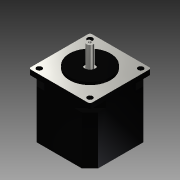
# Autodesk Inventor part: stepper
Saved by Autodesk Inventor 2015 SP1 (Build 190203100, 203)
## iProperties
Created: 2015-03-24
Part Number: stepper
Material: Ogólny
Document SubType Name: Modeling
Designer: Marcin
Density: 1 g/cm^3
Appearance: Gładki - czarny
Author: Marcin
Autodesk Inventor part; units mm, degrees
ref_plane "YZ Plane" through (0, 0, 0) normal (1, 0, 0) x (0, 1, 0)
ref_plane "XZ Plane" through (0, 0, 0) normal (0, 1, 0) x (-1, 0, 0)
ref_plane "XY Plane" through (0, 0, 0) normal (0, 0, 1) x (1, 0, 0)
sketch "Szkic1" plane through (0, 0, 0) normal (0, 0, 1) x (1, 0, 0)
  line L0 (-28.5, -28.5) -> (28.5, -28.5)
  line L1 (28.5, -28.5) -> (28.5, 28.5)
  line L2 (28.5, 28.5) -> (-28.5, 28.5)
  line L3 (-28.5, 28.5) -> (-28.5, -28.5)
  line L4 (-28.5, -28.5) -> (28.5, 28.5) construction
  line L5 (28.5, -28.5) -> (-28.5, 28.5) construction
  line L6 (-28.5, 20.9975) -> (-20.9975, 28.5)
  line L7 (20.9975, 28.5) -> (28.5, 20.9975)
  line L8 (28.5, -20.9975) -> (20.9975, -28.5)
  line L9 (-20.9975, -28.5) -> (-28.5, -20.9975)
  line L10 (0, 32.5269) -> (0, -32.5269) construction
  point P0 (0, 0)
  dimension "d0" = 57
  dimension "d3" = 70
  dimension "d4" = 70
  constraints: 22 end point, 8 point on line, 4 parallel, 3 midpoint, 3 perpendicular, 1 horizontal, 2 other
  measures "d0" distance of L0.end L1.end
  measures "d3" distance between parallel lines of L6 L8
  measures "d4" distance between parallel lines of L7 L9
extrude "Wyciągnięcie proste1" add sketch "Szkic1" along normal blind 45 contours L9 L3 L6 L2 L7 L1 L8 L0
sketch "Szkic2" plane through (0, 0, 45) normal (0, 0, 1) x (1, 0, 0)
  line L0 (20.9975, -28.5) -> (28.5, -20.9975) projected
  line L1 (28.5, -20.9975) -> (28.5, 20.9975) projected
  line L2 (28.5, 20.9975) -> (20.9975, 28.5) projected
  line L3 (20.9975, 28.5) -> (-20.9975, 28.5) projected
  line L4 (-20.9975, 28.5) -> (-28.5, 20.9975) projected
  line L5 (-28.5, 20.9975) -> (-28.5, -20.9975) projected
  line L6 (-28.5, -20.9975) -> (-20.9975, -28.5) projected
  line L7 (-20.9975, -28.5) -> (20.9975, -28.5) projected
  line L8 (20.9975, 28.5) -> (-20.9975, 28.5) projected
  line L9 (13.9264, 28.5) -> (28.5, 13.9264)
  line L10 (28.5, -20.9975) -> (28.5, 20.9975) projected
  line L11 (13.9264, -28.5) -> (28.5, -13.9264)
  line L12 (-20.9975, -28.5) -> (20.9975, -28.5) projected
  line L13 (-13.9264, -28.5) -> (-28.5, -13.9264)
  line L14 (-28.5, 20.9975) -> (-28.5, -20.9975) projected
  line L15 (-28.5, 13.9264) -> (-13.9264, 28.5)
  line L16 (-28.5, -20.9975) -> (-20.9975, -28.5) construction
  line L17 (-24.7487, -24.7487) -> (24.7487, 24.7487) construction
  line L18 (20.9975, -28.5) -> (28.5, -20.9975) construction
  line L19 (24.7487, -24.7487) -> (-24.7487, 24.7487) construction
  line L20 (-20.9975, 28.5) -> (-28.5, 20.9975) construction
  line L21 (-28.5, -20.9975) -> (-20.9975, -28.5) construction
  line L22 (28.5, 20.9975) -> (20.9975, 28.5) construction
  point P0 (0, 0)
  dimension "d7" = 60
  dimension "d8" = 60
  constraints: 12 end point, 8 point on line, 4 midpoint, 4 parallel, 2 other
  measures "d7" distance between parallel lines of L15 L11
  measures "d8" distance between parallel lines of L13 L9
extrude "Wyciągnięcie proste2" add sketch "Szkic2" along normal blind 6 contours L7 L13 L5 L15 L3 L9 L1 L11
sketch "Szkic3" plane through (0, 0, 51) normal (0, 0, 1) x (1, 0, 0)
  line L0 (20.9975, -28.5) -> (28.5, -20.9975) projected
  line L1 (-20.9975, -28.5) -> (20.9975, -28.5) projected
  line L2 (-28.5, -20.9975) -> (-20.9975, -28.5) projected
  line L3 (-28.5, 20.9975) -> (-28.5, -20.9975) projected
  line L4 (-20.9975, 28.5) -> (-28.5, 20.9975) projected
  line L5 (20.9975, 28.5) -> (-20.9975, 28.5) projected
  line L6 (28.5, 20.9975) -> (20.9975, 28.5) projected
  line L7 (28.5, -20.9975) -> (28.5, 20.9975) projected
  line L8 (-28.5, -28.5) -> (28.5, -28.5)
  line L9 (28.5, -28.5) -> (28.5, 28.5)
  line L10 (28.5, 28.5) -> (-28.5, 28.5)
  line L11 (-28.5, 28.5) -> (-28.5, -28.5)
  point P0 (0, 0)
  point P1 (0, 28.5)
  point P2 (28.5, 0)
  point P3 (0, -28.5)
  constraints: 8 end point, 6 midpoint, 2 parallel, 2 perpendicular, 1 horizontal
extrude "Wyciągnięcie proste3" add sketch "Szkic3" along normal blind 4.8
sketch "Szkic4" plane through (0, 0, 55.8) normal (0, 0, 1) x (1, 0, 0)
  circle A0 centre (0, 0) radius 19.05
  dimension "d13" = 38.1
  constraints: 1 centre point, 1 coincident
  measures "d13" diameter of A0
extrude "Wyciągnięcie proste4" add sketch "Szkic4" along normal blind 2.5
sketch "Szkic5" plane through (0, 0, 55.8) normal (0, 0, 1) x (1, 0, 0)
  line L0 (-23.57, -23.57) -> (23.57, -23.57) construction
  line L1 (23.57, -23.57) -> (23.57, 23.57) construction
  line L2 (23.57, 23.57) -> (-23.57, 23.57) construction
  line L3 (-23.57, 23.57) -> (-23.57, -23.57) construction
  line L4 (-23.57, -23.57) -> (23.57, 23.57) construction
  line L5 (23.57, -23.57) -> (-23.57, 23.57) construction
  point P0 (0, 0)
  dimension "d16" = 47.14
  constraints: 12 end point, 4 coincident, 2 midpoint, 2 parallel, 2 perpendicular, 1 horizontal
  measures "d16" distance of L0.end L1.end
hole "Otwór1" at (-23.57, 23.57, 55.8) at (23.57, 23.57, 55.8) at (23.57, -23.57, 55.8) at (-23.57, -23.57, 55.8) direction (0, 0, -1) diameter 5 depth 5
sketch "Szkic6" plane through (0, 0, 58.3) normal (0, 0, 1) x (1, 0, 0)
  circle A0 centre (0, 0) radius 5
  dimension "d24" = 10
  constraints: 1 centre point, 1 coincident
  measures "d24" diameter of A0
extrude "Wyciągnięcie proste5" cut sketch "Szkic6" against normal up to surface (2.5 mm away)
sketch "Szkic7" plane through (0, 0, 55.8) normal (0, 0, 1) x (1, 0, 0)
  circle A0 centre (0, 0) radius 5 projected
  circle A1 centre (0, 0) radius 3.175
  dimension "d27" = 6.35
  constraints: 1 centre point, 1 coincident
  measures "d27" diameter of A1
extrude "Wyciągnięcie proste6" add sketch "Szkic7" along normal blind 21 contours A1
sketch "Szkic8" plane through (0, 0, 76.8) normal (0, 0, 1) x (1, 0, 0)
  circle A0 centre (0, 0) radius 3.175 projected
  line L0 (-2.4659, 2) -> (2.4659, 2)
  dimension "d30" = 2
  constraints: 2 end point, 2 point on circle, 1 horizontal
  measures "d30" distance from line of L0 A0.centre
extrude "Wyciągnięcie proste7" cut sketch "Szkic8" against normal blind 19 contours L0 A0 picked at (-0.6547, 2.1648)
sketch "Szkic9" plane through (0, 0, 76.8) normal (0, 0, 1) x (1, 0, 0)
  point P0 (0, 0)
  point P1 (0, 0)
  constraints: 1 coincident
hole "Otwór2" at (0, 0, 76.8) direction (0, 0, -1) diameter 2.5 depth 2 tip angle 118
fillet "Zaokrąglenie1" radius 2 4 edges at (28.5, -28.5, 53.4) (28.5, 28.5, 53.4) (-28.5, 28.5, 53.4) (-28.5, -28.5, 53.4)
